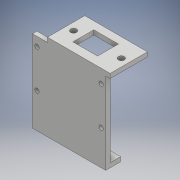
# Autodesk Inventor part: SoporteEthernet
Saved by Autodesk Inventor 2017 (Build 210142000, 142)
## iProperties
Created: 2021-08-13
Part Number: SoporteEthernet
Material: Generic
Document SubType Name: Modeling
Designer: USUARIO
Density: 1 g/cm^3
Appearance: Default
Author: USUARIO
Autodesk Inventor part; units mm, degrees
ref_plane "YZ Plane" through (0, 0, 0) normal (1, 0, 0) x (0, 1, 0)
ref_plane "XZ Plane" through (0, 0, 0) normal (0, 1, 0) x (-1, 0, 0)
ref_plane "XY Plane" through (0, 0, 0) normal (0, 0, 1) x (1, 0, 0)
sketch "Sketch1" plane through (0, 0, 0) normal (0, 1, 0) x (-1, 0, 0)
  line L0 (0, 0) -> (39, 0)
  line L1 (39, 0) -> (39, -51.8)
  line L2 (39, -51.8) -> (0, -51.8)
  line L3 (0, -51.8) -> (0, 0)
  dimension "d0" = 39
  dimension "d1" = 51.8
  constraints: 8 end point, 2 parallel, 1 horizontal, 1 perpendicular
  measures "d0" distance of L1.end L2.end
  measures "d1" distance of L0.end L1.end
extrude "Extrusion1" add sketch "Sketch1" along normal blind 3
sketch "Sketch2" plane through (-39, 0, 0) normal (0, 0, 1) x (1, 0, 0)
  line L0 (0, 0) -> (30, 0)
  line L1 (30, 0) -> (30, 25)
  line L2 (30, 25) -> (0, 25)
  line L3 (0, 25) -> (0, 0)
  point P0 (39, 0)
  dimension "d4" = 25
  constraints: 8 end point, 2 parallel, 1 horizontal, 1 perpendicular
  measures "d4" distance of L1.end L0.end
extrude "Extrusion2" add sketch "Sketch2" along normal blind 3
sketch "Sketch3" plane through (-39, 0, 3) normal (0, 0, 1) x (1, 0, 0)
  line L0 (11.25, 19.8) -> (27.75, 19.8)
  line L1 (27.75, 19.8) -> (27.75, 5.8)
  line L2 (27.75, 5.8) -> (11.25, 5.8)
  line L3 (11.25, 5.8) -> (11.25, 19.8)
  line L4 (0, 0) -> (39, 0) projected
  line L5 (30, 0) -> (30, 25) projected
  dimension "d7" = 16.5
  dimension "d8" = 14
  dimension "d9" = 5.8
  dimension "d10" = 2.25
  constraints: 8 end point, 2 parallel, 1 horizontal, 1 perpendicular
  measures "d7" distance of L1.end L2.end
  measures "d8" distance of L0.end L1.end
  measures "d9" distance between parallel lines of L4 L2
  measures "d10" distance between parallel lines of L5 L1
extrude "Extrusion3" cut sketch "Sketch3" against normal blind 3
sketch "Sketch5" plane through (-9, 3, 0) normal (1, 0, 0) x (0, 0, -1)
  line L0 (-3, -3) -> (-3, 22) projected
  line L1 (0, 0) -> (0, 22) projected
  line L2 (-3, -3) -> (0, -3)
  line L3 (0, -3) -> (0, 22)
  line L4 (0, 22) -> (-3, 22)
  line L5 (-3, 22) -> (-3, -3)
  point P0 (0, -3)
  constraints: 8 end point, 2 parallel, 1 horizontal, 1 perpendicular
extrude "Extrusion4" add sketch "Sketch5" along normal blind 12
sketch "Sketch6" plane through (-39, 0, 3) normal (0, 0, 1) x (1, 0, 0)
  circle A0 centre (5, 12.5) radius 2
  circle A1 centre (37, 12.5) radius 2
  line L0 (0, 25) -> (0, 0) projected
  line L1 (42, 25) -> (42, 0) projected
  line L2 (0, 25) -> (42, 25) projected
  point P0 (39, 0)
  dimension "d15" = 4
  dimension "d16" = 4
  dimension "d17" = 5
  dimension "d18" = 5
  dimension "d19" = 12.5
  dimension "d20" = 12.5
  constraints: 2 centre point
  measures "d15" diameter of A0
  measures "d16" diameter of A1
  measures "d17" distance from line of L0 A0.centre
  measures "d18" distance from line of L1 A1.centre
  measures "d19" distance from line of L2 A0.centre
  measures "d20" distance from line of L2 A1.centre
extrude "Extrusion5" cut sketch "Sketch6" against normal blind 9
sketch "Sketch7" plane through (-39, 0, -51.8) normal (-1, 0, 0) x (0, 0, 1)
  line L0 (0, 0) -> (0, 3) projected
  line L1 (0, 3) -> (51.8, 3)
  line L2 (51.8, 3) -> (51.8, 0)
  line L3 (51.8, 0) -> (0, 0)
  line L4 (0, 0) -> (0, 3)
  constraints: 8 end point, 2 parallel, 1 horizontal, 1 perpendicular
extrude "Extrusion6" add sketch "Sketch7" along normal blind 10
sketch "Sketch8" plane through (0, 3, 0) normal (0, 1, 0) x (1, 0, 0)
  circle A0 centre (-3, 31.478) radius 1.45
  circle A1 centre (-3, 6) radius 1.45
  circle A2 centre (-46, 31.4782) radius 1.45
  circle A3 centre (-46, 6) radius 1.45
  line L0 (0, 0) -> (0, 51.8) projected
  line L1 (-49, 0) -> (-49, 51.8) projected
  line L2 (-39, 0) -> (0, 0) projected
  line L3 (-39, 0) -> (-49, 0) projected
  dimension "d25" = 2.9
  dimension "d26" = 2.9
  dimension "d27" = 2.9
  dimension "d28" = 2.9
  dimension "d29" = 3
  dimension "d30" = 3
  dimension "d31" = 3
  dimension "d32" = 3
  dimension "d38" = 6
  dimension "d39" = 25.4782
  dimension "d40" = 25.478
  dimension "d41" = 6
  constraints: 4 centre point
  measures "d25" diameter of A0
  measures "d26" diameter of A1
  measures "d27" diameter of A2
  measures "d28" diameter of A3
  measures "d29" distance from line of A0.centre L0
  measures "d30" distance from line of A1.centre L0
  measures "d31" distance from line of A2.centre L1
  measures "d32" distance from line of A3.centre L1
  measures "d38" distance from line of L2 A1.centre
  measures "d39" distance of A2.centre A3.centre
  measures "d40" distance of A0.centre A1.centre
  measures "d41" distance from line of L3 A3.centre
extrude "Extrusion7" cut sketch "Sketch8" against normal blind 10
sketch "Sketch10" plane through (0, 0, -51.8) normal (0, 0, -1) x (-1, 0, 0)
  line L0 (-3, 25) -> (-3, 0) projected
  line L1 (0, 0) -> (49, 0)
  line L2 (49, 0) -> (49, 10)
  line L3 (49, 10) -> (0, 10)
  line L4 (0, 10) -> (0, 0)
  dimension "d35" = 10
  constraints: 8 end point, 2 parallel, 1 horizontal, 1 perpendicular
  measures "d35" distance of L2.end L1.end
extrude "Extrusion8" add sketch "Sketch10" along normal blind 3
body "Solid1"
